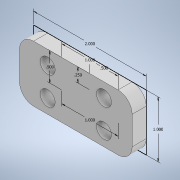
# Autodesk Inventor part: WellPlateFrame-AssemblyClip
Saved by Autodesk Inventor 2020 (Build 240168000, 168)
## iProperties
Created: 2023-02-23
Part Number: WellPlateFrame-AssemblyClip
Material: Generic
Document SubType Name: Modeling
Designer: Beaucage
Density: 1 g/cm^3
Appearance: Default
Author: Beaucage
Autodesk Inventor part; units mm, degrees
ref_plane "YZ Plane" through (0, 0, 0) normal (1, 0, 0) x (0, 1, 0)
ref_plane "XZ Plane" through (0, 0, 0) normal (0, 1, 0) x (-1, 0, 0)
ref_plane "XY Plane" through (0, 0, 0) normal (0, 0, 1) x (1, 0, 0)
sketch "Sketch1" plane through (0, 0, 0) normal (0, 0, 1) x (1, 0, 0)
  line L0 (0, 0) -> (50.8, 0)
  line L1 (50.8, 0) -> (50.8, 25.4)
  line L2 (50.8, 25.4) -> (0, 25.4)
  line L3 (0, 25.4) -> (0, 0)
  line L4 (25.4, 12.7) -> (25.4, 19.05)
  line L5 (25.4, 19.05) -> (38.1, 19.05)
  line L6 (38.1, 19.05) -> (12.7, 19.05)
  line L7 (12.7, 19.05) -> (12.7, 6.35)
  line L8 (12.7, 6.35) -> (38.1, 6.35)
  dimension "d0" = 50.8
  dimension "d1" = 25.4
  dimension "d2" = 6.35
  dimension "d3" = 12.7
  dimension "d4" = 25.4
  dimension "d5" = 12.7
  dimension "d6" = 25.4
  constraints: 18 end point, 4 perpendicular, 2 parallel, 1 horizontal, 1 point on line, 1 vertical
  measures "d0" distance of L2.end L1.end
  measures "d1" distance of L1.end L0.end
  measures "d2" distance of L4.start L4.end
  measures "d3" distance of L4.end L5.end
  measures "d4" distance of L5.end L6.end
  measures "d5" distance of L6.end L7.end
  measures "d6" distance of L7.end L8.end
extrude "Extrusion1" add sketch "Sketch1" along normal blind 6.35
hole "Hole1" at (38.1, 19.05, 0) at (38.1, 6.35, 0) at (12.7, 6.35, 0) at (12.7, 19.05, 0) direction (0, 0, 1) diameter 6.7564 end through all clearance for "Socket Head Cap Screw" size "1/4" standard "Ansi Unified Screw Threads"
fillet "Fillet1" radius 6.35 4 edges at (50.8, 25.4, 3.175) (50.8, 0, 3.175) (0, 25.4, 3.175) (0, 0, 3.175)
body "Solid1"
